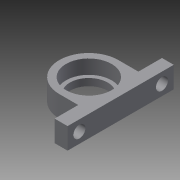
# Autodesk Inventor part: wheel_shaft_holder_small
Saved by Autodesk Inventor 2015 (Build 190159000, 159)
## iProperties
Created: 2017-12-14
Part Number: wheel_shaft_holder_small
Material: Generic
Document SubType Name: Modeling
Designer: Anshul
Density: 1 g/cm^3
Appearance: Default
Author: Anshul
Autodesk Inventor part; units mm, degrees
ref_plane "YZ Plane" through (0, 0, 0) normal (1, 0, 0) x (0, 1, 0)
ref_plane "XZ Plane" through (0, 0, 0) normal (0, 1, 0) x (-1, 0, 0)
ref_plane "XY Plane" through (0, 0, 0) normal (0, 0, 1) x (1, 0, 0)
sketch "Sketch1" plane through (0, 0, 0) normal (0, 1, 0) x (-1, 0, 0)
  line L0 (0, 0) -> (12.5, 0)
  circle A0 centre (12.5, 0) radius 9.65
  circle A1 centre (12.5, 0) radius 12.5
  line L1 (12.5, 12.5) -> (-1, 12.5)
  line L2 (-1, 12.5) -> (-1, -12.5)
  line L3 (-1, -12.5) -> (12.5, -12.5)
  circle A2 centre (12.5, 0) radius 8
  line L4 (-1, -12.5) -> (4, -12.5)
  line L5 (4, -12.5) -> (4, -22.5)
  line L6 (4, -22.5) -> (-1, -22.5)
  line L7 (-1, -22.5) -> (-1, -12.5)
  line L8 (-1, 12.5) -> (-1, 22.5)
  line L9 (-1, 22.5) -> (4.5, 22.5)
  line L10 (4.5, 22.5) -> (4.5, 12.5)
  dimension "d0" = 12.5
  dimension "d1" = 19.3
  dimension "d2" = 16
  dimension "d7" = 5
  dimension "d8" = 10
  dimension "d9" = 10
  constraints: 22 end point, 5 perpendicular, 3 centre point, 3 coincident, 3 point on circle, 3 point on line, 2 horizontal, 2 tangent, 1 collinear
  measures "d0" distance of L0.start L0.end
  measures "d1" diameter of A0
  measures "d2" diameter of A2
  measures "d7" distance of L2.end L4.end
  measures "d8" distance of L4.end L5.end
  measures "d9" distance of L1.end L8.end
extrude "Extrusion3" add sketch "Sketch1" along normal blind 3 contours A0
extrude "Extrusion4" add sketch "Sketch1" along normal blind 9 contours A1 L3 L2 L1 | A1 | L1 L8 L9 L10 | L5 L6 L7 L3
sketch "Sketch4" plane through (1, 0, 22.5) normal (1, 0, 0) x (0, 0, -1)
  line L0 (0, 0) -> (0, 9) projected
  line L1 (0, 4.5) -> (5, 4.5)
  line L2 (45, 0) -> (45, 9) projected
  line L3 (45, 4.5) -> (40, 4.5)
  circle A0 centre (5, 4.5) radius 2.55
  circle A1 centre (40, 4.5) radius 2.55
  point P0 (22.5, 0)
  dimension "d14" = 5
  dimension "d15" = 5
  dimension "d16" = 5.1
  dimension "d17" = 5.1
  constraints: 4 end point, 2 centre point, 2 coincident, 2 midpoint, 1 horizontal, 1 point on line
  measures "d14" distance of L1.start L1.end
  measures "d15" distance of L3.start L3.end
  measures "d16" diameter of A0
  measures "d17" diameter of A1
extrude "Extrusion5" cut sketch "Sketch4" against normal blind 7
body "Solid2"
